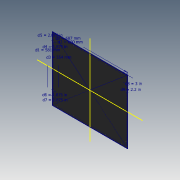
# Autodesk Inventor part: Standard
Saved by Autodesk Inventor 2020.3 (Build 243373000, 373)
## iProperties
RuleStatus: InUse
AfterDocSave0: file://Part Number Cleaner
Created: 2023-02-14
Material: ACRYLIC, BLACK
Catalog Web Link: https://www.janelia.org/
Vendor: HHMI: JRC - jET
Document SubType Name: Modeling
Designer: arnoldj
Density: 1 g/cm^3
Appearance: Generic
DESIGN DEPARTMENT: HHMI: JRC - jET
ALTERED ITEM PART NUMBER: N/A
ALTERED ITEM VENDOR: N/A
ALTERED ITEM DESCRIPTION: N/A
Title: Standard
Author: arnoldj
Revision Number: 0
Autodesk Inventor part; units mm, degrees
ref_plane "YZ Plane" through (0, 0, 0) normal (1, 0, 0) x (0, 1, 0)
ref_plane "XZ Plane" through (0, 0, 0) normal (0, 1, 0) x (-1, 0, 0)
ref_plane "XY Plane" through (0, 0, 0) normal (0, 0, 1) x (1, 0, 0)
sketch "Sketch1" plane through (0, 0, 0) normal (0, 0, 1) x (1, 0, 0)
  line L0 (0, 406.7) -> (0, -406.7) projected
  line L1 (-480.9, 0) -> (480.9, 0) projected
  line L2 (343.5, -290.5) -> (-343.5, -290.5)
  line L3 (-343.5, -290.5) -> (-343.5, 290.5)
  line L4 (-343.5, 290.5) -> (343.5, 290.5)
  line L5 (343.5, 290.5) -> (343.5, -290.5)
  line L6 (343.5, -290.5) -> (-343.5, 290.5) construction
  line L7 (-343.5, -290.5) -> (343.5, 290.5) construction
  line L8 (330, -277) -> (-330, -277) construction
  line L9 (-330, -277) -> (-330, 277) construction
  line L10 (-330, 277) -> (330, 277) construction
  line L11 (330, 277) -> (330, -277) construction
  line L12 (330, -277) -> (-330, 277) construction
  line L13 (-330, -277) -> (330, 277) construction
  point P0 (0, 0)
  point P1 (-330, 217.475)
  point P2 (-330, 169.85)
  point P3 (-330, -217.475)
  point P4 (-330, -169.85)
  point P5 (330, 214.3)
  point P6 (330, 158.42)
  dimension "d0" = 687
  dimension "d1" = 581
  dimension "d2" = 660
  dimension "d3" = 554
  dimension "d4" = 47.625
  dimension "d5" = 73.025
  dimension "d6" = 47.625
  dimension "d7" = 73.025
  dimension "d8" = 76.2
  dimension "d9" = 55.88
  constraints: 24 end point, 6 point on line, 4 midpoint, 4 parallel, 2 horizontal, 2 perpendicular
  measures "d0" distance of L3.end L4.end
  measures "d1" distance of L2.end L3.end
  measures "d2" distance of L9.end L10.end
  measures "d3" distance of L8.end L9.end
  measures "d4" distance of point (-330, 169.85) point (-330, 217.475)
  measures "d5" distance from line of point (-330, 217.475) L4
  measures "d6" distance of point (-330, -217.475) point (-330, -169.85)
  measures "d7" distance from line of point (-330, -217.475) L2
  measures "d8" distance from line of point (330, 214.3) L4
  measures "d9" distance of point (330, 214.3) point (330, 158.42)
extrude "Extrusion1" add sketch "Sketch1" against normal blind 3.175
hole "Hole1" at (-330, 217.475, 0) at (-330, 169.85, 0) at (-330, -217.475, 0) at (-330, -169.85, 0) at (330, 214.3, 0) at (330, 158.42, 0) direction (0, 0, -1) diameter 6.096 end through all
sketch "Sketch2" plane through (0, 0, 0) normal (0, 0, 1) x (1, 0, 0)
  line L0 (-330, -277) -> (-330, 277) construction
  line L1 (-330, 277) -> (330, 277) construction
  line L2 (330, 277) -> (330, -277) construction
  line L3 (330, -277) -> (-330, -277) construction
  line L4 (0, 406.7) -> (0, -406.7) projected
  line L5 (-480.9, 0) -> (480.9, 0) projected
  point P0 (0, 0)
  point P1 (-330, 241.3)
  point P2 (-292.1, 277)
  point P3 (292.1, 277)
  point P4 (0, 277)
  point P5 (-146.05, 277)
  point P6 (146.05, 277)
  point P7 (330, 241.3)
  point P8 (330, 120.65)
  point P9 (330, 0)
  point P10 (330, -120.65)
  point P11 (292.1, -277)
  point P12 (146.05, -277)
  point P13 (0, -277)
  point P14 (-146.05, -277)
  point P15 (-292.1, -277)
  point P16 (-330, -241.3)
  point P17 (-330, -120.65)
  point P18 (-330, 0)
  point P19 (-330, 120.65)
  point P20 (330, -241.3)
  dimension "d19" = 146.05
  dimension "d20" = 146.05
  dimension "d21" = 146.05
  dimension "d22" = 146.05
  dimension "d23" = 120.65
  dimension "d24" = 120.65
  dimension "d25" = 120.65
  dimension "d26" = 120.65
  constraints: 16 point on line, 4 horizontal alignment, 4 midpoint, 4 vertical alignment
  measures "d19" distance from line of L4 point (-146.05, 277)
  measures "d20" distance from line of point (146.05, 277) L4
  measures "d21" distance of point (146.05, 277) point (292.1, 277)
  measures "d22" distance of point (-146.05, 277) point (-292.1, 277)
  measures "d23" distance from line of L5 point (-330, 120.65)
  measures "d24" distance from line of point (-330, -120.65) L5
  measures "d25" distance of point (-330, 120.65) point (-330, 241.3)
  measures "d26" distance of point (-330, -120.65) point (-330, -241.3)
hole "Hole2" at (-292.1, 277, 0) at (-146.05, 277, 0) at (146.05, 277, 0) at (292.1, 277, 0) at (330, 0, 0) at (330, -241.3, 0) at (292.1, -277, 0) at (146.05, -277, 0) at (0, -277, 0) at (-146.05, -277, 0) at (-292.1, -277, 0) at (-330, 0, 0) at (0, 277, 0) direction (0, 0, -1) diameter 4.572 end through all
fillet "Fillet1" radius 4.7625 4 edges at (343.5, 290.5, -1.5875) (-343.5, 290.5, -1.5875) (343.5, -290.5, -1.5875) (-343.5, -290.5, -1.5875)
body "Solid1"
